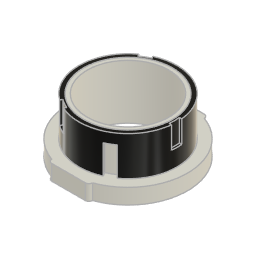
Soundwell EC350302X2A-HA1 (Autodesk Fusion 360 design; units mm, degrees)
Autodesk Fusion 360 part; units mm, degrees
sketch "Sketch1" plane through (0, 0, 0) normal (0, 0, 1) x (1, 0, 0)
  line L0 (-4.9393, 17.5) -> (4.9393, 17.5)
  arc A0 (17.5, 0) -> (6, 16.4393) centre (0, 0) ccw
  arc A1 (-6, 16.4393) -> (-17.5, 0) centre (0, 0) ccw
  arc A2 (-4.9393, 17.5) -> (-6, 16.4393) centre (-4.9393, 16.4393) ccw
  arc A3 (6, 16.4393) -> (4.9393, 17.5) centre (4.9393, 16.4393) ccw
  line L1 (-17.5, 0) -> (17.5, 0) construction
  arc A4 (-17.5, 0) -> (-6, -16.4393) centre (0, 0) ccw
  arc A5 (-6, -16.4393) -> (-4.9393, -17.5) centre (-4.9393, -16.4393) ccw
  line L2 (-4.9393, -17.5) -> (4.9393, -17.5)
  arc A6 (4.9393, -17.5) -> (6, -16.4393) centre (4.9393, -16.4393) ccw
  arc A7 (6, -16.4393) -> (17.5, 0) centre (0, 0) ccw
  circle A8 centre (0, 0) radius 12.7
  dimension "d2" = 35
  dimension "d4" = 12
  dimension "d7" = 25.4
  constraint coincident A0.centre A1.centre
  constraint horizontal A0.centre A0.start
  constraint horizontal A0.centre A1.end
  constraint coincident A1.start A0
  constraint tangent L0 A0
  constraint concentric A0 A1
  constraint coincident A1.start A2.end
  constraint tangent L0 A2
  constraint horizontal L0
  constraint coincident A0.end A3.start
  constraint tangent L0 A3
  constraint equal A2 A3
  constraint horizontal A1.start A0.end
  constraint horizontal A1.start A2.centre
  constraint symmetric A0.start L1 A7.end
  constraint symmetric A1.end L1 A4.start
  constraint symmetric A1.start L1 A4.end
  constraint symmetric L0.end L1 L2.end
  constraint symmetric A0.end L1 A6.end
  constraint symmetric A0 L1 A7
  constraint symmetric A1 L1 A4
  constraint symmetric L0.start L1 A5.end
  constraint symmetric A2 L1 A5
  constraint symmetric A3 L1 A6
  constraint concentric A0 A8
  measures "d2" distance of A0.start A1.end
  measures "d4" horizontal distance of A1.start A0.end
  measures "d7" diameter of A8
extrude "Extrude1" add sketch "Sketch1" along normal blind 4.5 makes body 1
sketch "Sketch3" plane through (0, 0, 4.5) normal (0, 0, 1) x (1, 0, 0)
  circle A0 centre (0, 0) radius 14.4
  circle A1 centre (0, 0) radius 12.7
  arc A2 (-4.9393, 17.5) -> (-6, 16.4393) centre (-4.9393, 16.4393) ccw
  arc A3 (-6, 16.4393) -> (-6, -16.4393) centre (0, 0) ccw
  arc A4 (-6, -16.4393) -> (-4.9393, -17.5) centre (-4.9393, -16.4393) ccw
  line L0 (-4.9393, -17.5) -> (4.9393, -17.5)
  arc A5 (4.9393, -17.5) -> (6, -16.4393) centre (4.9393, -16.4393) ccw
  arc A6 (6, -16.4393) -> (6, 16.4393) centre (0, 0) ccw
  arc A7 (6, 16.4393) -> (4.9393, 17.5) centre (4.9393, 16.4393) ccw
  line L1 (4.9393, 17.5) -> (-4.9393, 17.5)
  circle A8 centre (0, 0) radius 13.1
  dimension "d8" = 28.8
  dimension "d9" = 1.3
  constraint coincident A0.centre A1.centre
  measures "d8" diameter of A0
  measures "d9" distance of A0 A8
extrude "Extrude2" add sketch "Sketch3" along normal blind 11.5 separate body contours A0 makes body 2
sketch "Sketch4" plane through (0, 0, 4.5) normal (0, 0, -1) x (1, 0, 0)
  circle A0 centre (0, 0) radius 13.1
  circle A1 centre (0, 0) radius 14.4
  line L0 (-14.3217, -1.5) -> (-13.0138, -1.5)
  line L1 (-13.0138, 1.5) -> (-14.3217, 1.5)
  line L2 (8.4599, -11.6529) -> (7.806, -10.5203)
  line L3 (5.2079, -12.0203) -> (5.8618, -13.1529)
  line L4 (5.8618, 13.1529) -> (5.2079, 12.0203)
  line L5 (7.806, 10.5203) -> (8.4599, 11.6529)
  dimension "d13" = 3
  dimension "d15" = 360
  constraint coincident A1 L0.start
  constraint coincident A0 L0.end
  constraint horizontal L0
  constraint coincident A0 L1.start
  constraint coincident A1 L1.end
  constraint horizontal L1
  constraint equal L0 L1
  measures "d13" distance of L0 L1
extrude "Extrude3" cut sketch "Sketch4" against normal blind 8.5 contours A0 A1 L4 L5 | A0 A1 L2 L3 | A0 A1 L0 L1 bodies 2
sketch "Sketch5" plane through (0, 0, 16) normal (0, 0, 1) x (-1, 0, 0)
  circle A0 centre (0, 0) radius 13.1
  circle A1 centre (0, 0) radius 14.4
  line L0 (-14.3217, 1.5) -> (-13.6176, 1.5)
  arc A2 (-13.6176, 1.5) -> (-13.6176, -1.5) centre (0, 0) ccw
  line L1 (-13.6176, -1.5) -> (-14.3217, -1.5)
  arc A3 (5.5098, -12.5432) -> (8.1079, -11.0432) centre (0, 0) ccw
  line L2 (8.1079, -11.0432) -> (8.4599, -11.6529)
  line L3 (5.8618, -13.1529) -> (5.5098, -12.5432)
  arc A4 (8.1079, 11.0432) -> (5.5098, 12.5432) centre (0, 0) ccw
  line L4 (5.5098, 12.5432) -> (5.8618, 13.1529)
  line L5 (8.4599, 11.6529) -> (8.1079, 11.0432)
  dimension "d18" = 3
  dimension "d19" = 0.7
  dimension "d21" = 360
  constraint coincident A1 L0.start
  constraint horizontal L0
  constraint coincident A0.centre A1.centre
  constraint coincident A1 L1.end
  constraint horizontal L1
  constraint vertical L0.end A2.end
  measures "d18" distance of L0 L1
  measures "d19" distance of A1 A2
extrude "Extrude4" cut sketch "Sketch5" against normal blind 6.5 contours A1 A4 L4 L5 | A1 A3 L2 L3 | A1 L0 A2 L1 bodies 2
sketch "Sketch6" plane through (0, 0, 0) normal (0, 0, 1) x (1, 0, 0)
  circle A0 centre (0, 0) radius 13.1
  circle A1 centre (0, 0) radius 12
  dimension "d26" = 24
  constraint concentric A0 A1
  measures "d26" diameter of A1
extrude "Extrude5" add sketch "Sketch6" along normal up to surface (16 mm away) bodies 1
sketch "Sketch7" plane through (0, 0, 0) normal (0, 0, -1) x (1, 0, 0)
  circle A0 centre (0, 0) radius 12
  arc A1 (-6, -16.4393) -> (-4.9393, -17.5) centre (-4.9393, -16.4393) ccw
  line L0 (-4.9393, -17.5) -> (4.9393, -17.5)
  arc A2 (4.9393, -17.5) -> (6, -16.4393) centre (4.9393, -16.4393) ccw
  arc A3 (6, -16.4393) -> (6, 16.4393) centre (0, 0) ccw
  arc A4 (6, 16.4393) -> (4.9393, 17.5) centre (4.9393, 16.4393) ccw
  line L1 (4.9393, 17.5) -> (-4.9393, 17.5)
  arc A5 (-4.9393, 17.5) -> (-6, 16.4393) centre (-4.9393, 16.4393) ccw
  arc A6 (-6, 16.4393) -> (-6, -16.4393) centre (0, 0) ccw
  circle A7 centre (-5.0277, -13.8135) radius 0.75
  line L2 (-5.0277, -13.8135) -> (5.0277, 13.8135) construction
  circle A8 centre (5.0277, 13.8135) radius 0.75
  line L3 (0, -1.75) -> (0, -22.5) construction
  dimension "d27" = 20
  dimension "d28" = 1.5
  dimension "d29" = 29.4
  constraint coincident A7.centre L2.start
  constraint coincident L2.end A8.centre
  constraint midpoint A0.centre L2
  constraint equal A7 A8
  measures "d27" angle of L2 L3
  measures "d28" diameter of A7
  measures "d29" distance of A7.centre L2.end
extrude "Extrude6" add sketch "Sketch7" along normal blind 1.5 contours A7 | A8 bodies 1
equation "d9 = 2.4 mm - 1.1 mm"
equation "d16 = 3 mm - 11.50 mm"
equation "d19 = 2.3 mm - 1.6 mm"
named bodies: "Wheel"
